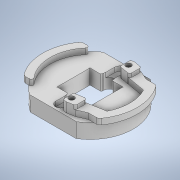
# Autodesk Inventor part: sketch01
Saved by Autodesk Inventor 2020 (Build 240168000, 168)
## iProperties
Created: 2024-03-18
Part Number: sketch01
Material: Типовые
Document SubType Name: Modeling
Designer: 4s
Density: 1 g/cm^3
Appearance: По умолчанию
Author: 4s
Autodesk Inventor part; units mm, degrees
ref_plane "YZ Plane" through (0, 0, 0) normal (1, 0, 0) x (0, 1, 0)
ref_plane "XZ Plane" through (0, 0, 0) normal (0, 1, 0) x (-1, 0, 0)
ref_plane "XY Plane" through (0, 0, 0) normal (0, 0, 1) x (1, 0, 0)
sketch "Эскиз1" plane through (0, 0, 0) normal (0, 1, 0) x (-1, 0, 0)
  line L0 (8.55, 8.55) -> (2.65, 8.55)
  line L1 (-8.55, 8.55) -> (-8.55, -8.55)
  line L2 (-8.55, -8.55) -> (-2.65, -8.55)
  line L3 (8.55, -8.55) -> (8.55, 8.55)
  line L4 (0, 0) -> (14.8515, 0) construction
  line L5 (0, 0) -> (0, -24.3542) construction
  line L6 (12.9542, 12.5) -> (-4.4938, 12.5) construction
  line L7 (12.9542, -12.5) -> (-4.4938, -12.5) construction
  arc A0 (2.65, 9.85) -> (-2.65, 9.85) centre (0, 9.85) ccw
  line L8 (2.65, 9.85) -> (2.65, 8.55)
  line L9 (-2.65, 9.85) -> (-2.65, 8.55)
  arc A1 (2.3092, 8.55) -> (2.65, 9.85) centre (0, 9.85) ccw construction
  arc A2 (-2.3092, 8.55) -> (2.3092, 8.55) centre (0, 9.85) ccw construction
  arc A3 (-2.65, 9.85) -> (-2.3092, 8.55) centre (0, 9.85) ccw construction
  line L10 (2.65, 8.55) -> (-2.65, 8.55) construction
  line L11 (-2.65, 8.55) -> (-8.55, 8.55)
  arc A4 (-2.65, -9.85) -> (2.65, -9.85) centre (0, -9.85) ccw
  line L12 (2.65, -9.85) -> (2.65, -8.55)
  line L13 (-2.65, -9.85) -> (-2.65, -8.55)
  arc A5 (2.65, -9.85) -> (2.3092, -8.55) centre (0, -9.85) ccw construction
  arc A6 (-2.3092, -8.55) -> (-2.65, -9.85) centre (0, -9.85) ccw construction
  line L14 (2.65, -8.55) -> (8.55, -8.55)
  line L15 (-2.65, -8.55) -> (2.65, -8.55) construction
  circle A7 centre (0, 0) radius 22.35
  dimension "d0" = 17.1
  dimension "d1" = 17.1
  dimension "d2" = 25
  dimension "d3" = 5.3
  dimension "d4" = 44.7
  constraints: 32 end point, 14 point on circle, 11 symmetric about line, 10 parallel, 8 centre point, 6 tangent, 5 horizontal, 5 point on line, 3 perpendicular, 2 vertical, 1 coincident, 5 other
  measures "d0" distance of L3.start L0.start
  measures "d1" distance of L1.end L3.start
  measures "d2" distance between parallel lines of L6 L7
  measures "d3" diameter of A0
  measures "d4" diameter of A7
extrude "Выдавливание1" add sketch "Эскиз1" along normal blind 7.7
sketch "Эскиз2" plane through (0, 7.7, 0) normal (0, 1, 0) x (1, 0, 0)
  line L0 (0, 0) -> (0, 23.6415) construction
  arc A0 (0, 12.825) -> (2.5, 15.325) centre (0, 15.325) ccw construction
  line L1 (0, 0) -> (14.5442, 0) construction
  arc A1 (-2.5, -15.325) -> (2.5, -15.325) centre (0, -15.325) ccw
  line L2 (2.5, -15.325) -> (2.5, -10.7289)
  circle A2 centre (0, 0) radius 22.35 construction
  line L3 (-8.55, 8.55) -> (-2.65, 8.55) construction
  line L4 (-2.65, 8.55) -> (-2.65, 9.85) construction
  arc A3 (2.65, 9.85) -> (-2.65, 9.85) centre (0, 9.85) ccw construction
  line L5 (2.65, 9.85) -> (2.65, 8.55) construction
  line L6 (2.65, 8.55) -> (8.55, 8.55) construction
  line L7 (8.55, 8.55) -> (8.55, -8.55) construction
  line L8 (8.55, -8.55) -> (2.65, -8.55) construction
  line L9 (2.65, -8.55) -> (2.65, -9.85) construction
  arc A4 (-2.65, -9.85) -> (2.65, -9.85) centre (0, -9.85) ccw construction
  line L10 (-2.65, -9.85) -> (-2.65, -8.55) construction
  line L11 (-2.65, -8.55) -> (-8.55, -8.55) construction
  line L12 (-8.55, -8.55) -> (-8.55, 8.55) construction
  line L13 (0, 0) -> (0, -9.85) construction
  line L14 (0, 0) -> (-8.55, 0) construction
  line L15 (-2.5, -15.325) -> (-2.5, -10.7289)
  line L16 (2.5, 15.325) -> (2.5, 10.7289)
  line L17 (-2.5, 15.325) -> (-2.5, 10.7289)
  arc A5 (2.5, -15.325) -> (-2.5, -15.325) centre (0, -15.325) ccw construction
  arc A6 (-2.5, 15.325) -> (0, 12.825) centre (0, 15.325) ccw construction
  arc A7 (2.5, 15.325) -> (-2.5, 15.325) centre (0, 15.325) ccw
  line L18 (2.5, -10.7289) -> (-2.5, -10.7289)
  line L19 (2.5, 10.7289) -> (-2.5, 10.7289)
  dimension "d7" = 5
  dimension "d8" = 30.65
  constraints: 20 end point, 11 point on circle, 7 symmetric about line, 5 centre point, 3 horizontal, 3 vertical, 2 point on line, 1 midpoint, 1 tangent, 1 other
  measures "d7" diameter of A0
  measures "d8" distance of A1.centre A0.centre
extrude "Выдавливание2" cut sketch "Эскиз2" against normal blind 2.5
ref_plane "РабПлоскость1" through (0, 0, -8.55) normal (-1, 0, 0) x (0, 0, 1)
sketch "Эскиз3" plane through (0, 0, -8.55) normal (-1, 0, 0) x (0, 0, 1)
  line L0 (30.9, 7.7) -> (-13.8, 7.7) construction
  line L1 (30.9, 0) -> (-13.8, 0) construction
  line L2 (30.9, 0) -> (-13.8, 0) construction
  line L3 (30.9, 0) -> (31.1, 7.7)
  line L4 (30.9, 7.7) -> (-13.8, 7.7) construction
  line L5 (31.1, 7.7) -> (30.9, 7.7)
  line L6 (30.9, 7.7) -> (30.9, 0)
  line L7 (30.9, 0) -> (30.9, 7.7) construction
  line L8 (8.55, -1.54) -> (8.55, 9.24) projected
  point P0 (8.55, 0)
  dimension "d11" = 0.2
  constraints: 6 end point, 1 collinear, 1 horizontal, 1 point on line
  measures "d11" distance of L3.end L0.start
revolve "Вращение1" add sketch "Эскиз3" angle 360 about axis through (0, 0, 0) along (0, 1, 0)
sketch "Эскиз4" plane through (0, 7.7, 0) normal (0, 1, 0) x (1, 0, 0)
  circle A0 centre (0, 0) radius 22.55 construction
  line L0 (2.5, 15.325) -> (2.5, 10.7289) construction
  arc A1 (2.65, 9.85) -> (2.5, 10.7289) centre (0, 9.85) ccw construction
  line L1 (2.65, 9.85) -> (2.65, 8.55) construction
  line L2 (2.65, 8.55) -> (8.55, 8.55) construction
  line L3 (8.55, 8.55) -> (8.55, -8.55) construction
  line L4 (8.55, -8.55) -> (2.65, -8.55) construction
  line L5 (2.65, -8.55) -> (2.65, -9.85) construction
  arc A2 (2.5, -10.7289) -> (2.65, -9.85) centre (0, -9.85) ccw construction
  line L6 (2.5, -10.7289) -> (2.5, -15.325) construction
  arc A3 (-2.5, -15.325) -> (2.5, -15.325) centre (0, -15.325) ccw construction
  line L7 (-2.5, -15.325) -> (-2.5, -10.7289) construction
  arc A4 (-2.65, -9.85) -> (-2.5, -10.7289) centre (0, -9.85) ccw construction
  line L8 (-2.65, -9.85) -> (-2.65, -8.55) construction
  line L9 (-2.65, -8.55) -> (-8.55, -8.55) construction
  line L10 (-8.55, -8.55) -> (-8.55, 8.55) construction
  line L11 (-8.55, 8.55) -> (-2.65, 8.55) construction
  line L12 (-2.65, 8.55) -> (-2.65, 9.85) construction
  arc A5 (-2.5, 10.7289) -> (-2.65, 9.85) centre (0, 9.85) ccw construction
  line L13 (-2.5, 10.7289) -> (-2.5, 15.325) construction
  arc A6 (2.5, 15.325) -> (-2.5, 15.325) centre (0, 15.325) ccw construction
  circle A7 centre (0, 0) radius 24.4 construction
  line L14 (-25.2679, -15) -> (28.9131, -15) construction
  line L15 (0, 0) -> (22.55, 0) construction
  line L16 (-25.2679, 15) -> (28.9131, 15) construction
  arc A8 (-19.2447, 15) -> (-19.2447, -15) centre (0, 0) ccw
  circle A9 centre (0, 0) radius 22.55 construction
  arc A10 (-16.8375, 15) -> (-16.8375, -15) centre (0, 0) ccw
  line L17 (-16.8375, 15) -> (-19.2447, 15)
  line L18 (-16.8375, -15) -> (-19.2447, -15)
  line L19 (0, 0) -> (0, 9.85) construction
  arc A11 (19.2447, -15) -> (19.2447, 15) centre (0, 0) ccw
  arc A12 (16.8375, -15) -> (16.8375, 15) centre (0, 0) ccw
  line L20 (16.8375, 15) -> (19.2447, 15)
  line L21 (16.8375, -15) -> (19.2447, -15)
  circle A13 centre (0, 0) radius 20.55 construction
  arc A14 (-14.0464, 15) -> (-14.0464, -15) centre (0, 0) ccw
  line L22 (-16.8375, -15) -> (-14.0464, -15)
  line L23 (-16.8375, 15) -> (-14.0464, 15)
  arc A15 (16.8375, -15) -> (16.8375, 15) centre (0, 0) ccw
  arc A16 (14.0464, -15) -> (14.0464, 15) centre (0, 0) ccw
  line L24 (16.8375, -15) -> (14.0464, -15)
  line L25 (16.8375, 15) -> (14.0464, 15)
  dimension "d13" = 1.85
  dimension "d14" = 30
  dimension "d15" = 2
  constraints: 24 end point, 20 point on circle, 9 centre point, 8 symmetric about line, 6 point on line, 4 collinear, 3 coincident, 2 concentric, 2 horizontal, 1 horizontal alignment, 1 vertical, 5 other
  measures "d14" distance between parallel lines of L14 L16
  measures "d15" radial gap between concentric circles of A9 A13
extrude "Выдавливание3" add sketch "Эскиз4" along normal blind 3
sketch "Эскиз5" plane through (0, 7.7, 0) normal (0, 1, 0) x (1, 0, 0)
  line L0 (-19.0815, -19) -> (24.7344, -19)
  line L1 (0, 0) -> (-21.0145, 0) construction
  line L2 (-19.0815, 19) -> (24.7344, 19)
  line L3 (-19.0815, -19) -> (0, -30.6052)
  line L4 (0, -30.6052) -> (24.7344, -19)
  line L5 (-19.0815, 19) -> (0, 30.6052)
  line L6 (0, 30.6052) -> (24.7344, 19)
  dimension "d18" = 38
  constraints: 14 end point, 3 symmetric about line, 2 horizontal
  measures "d18" distance between parallel lines of L0 L2
extrude "Выдавливание4" cut sketch "Эскиз5" against normal blind 10
sketch "Эскиз6" plane through (0, 0, 0) normal (0, -1, 0) x (1, 0, 0)
  line L0 (-8.55, -8.55) -> (-2.65, -8.55) construction
  line L1 (-8.55, 8.55) -> (-8.55, -8.55) construction
  line L2 (-2.65, 8.55) -> (-8.55, 8.55) construction
  line L3 (-2.65, 9.85) -> (-2.65, 8.55) construction
  arc A0 (2.65, 9.85) -> (-2.65, 9.85) centre (0, 9.85) ccw construction
  line L4 (2.65, 8.55) -> (2.65, 9.85) construction
  line L5 (8.55, 8.55) -> (2.65, 8.55) construction
  line L6 (8.55, -8.55) -> (8.55, 8.55) construction
  line L7 (2.65, -8.55) -> (8.55, -8.55) construction
  line L8 (2.65, -9.85) -> (2.65, -8.55) construction
  arc A1 (-2.65, -9.85) -> (2.65, -9.85) centre (0, -9.85) ccw construction
  line L9 (-2.65, -8.55) -> (-2.65, -9.85) construction
  line L10 (11.7696, 19) -> (-11.7696, 19) construction
  arc A2 (-11.7696, 19) -> (-11.7696, -19) centre (0, 0) ccw construction
  line L11 (-11.7696, -19) -> (11.7696, -19) construction
  arc A3 (11.7696, -19) -> (11.7696, 19) centre (0, 0) ccw construction
  line L12 (0, 9.85) -> (0, -9.85) construction
  line L13 (5.2, 15.6144) -> (5.2, -19.2684) construction
  circle A4 centre (5.2, 14.73) radius 3
  line L14 (0, 0) -> (12.7477, 0) construction
  circle A5 centre (5.2, -14.73) radius 3
  dimension "d21" = 5.2
  dimension "d22" = 6
  dimension "d23" = 29.46
  constraints: 6 end point, 2 centre point, 1 horizontal, 1 parallel, 1 point on line, 1 symmetric about line, 1 vertical, 1 other
  measures "d21" distance between parallel lines of L12 L13
  measures "d22" diameter of A4
  measures "d23" distance of A5.centre A4.centre
extrude "Выдавливание5" cut sketch "Эскиз6" against normal blind 10
sketch "Эскиз7" plane through (0, 0, 0) normal (0, -1, 0) x (1, 0, 0)
  line L0 (0, 0) -> (0, -17.2955) construction
  line L1 (9.5, 17) -> (9.5, -18.6283) construction
  line L2 (9.5, 17) -> (15.5, 13.5359)
  circle A0 centre (5.2, -14.73) radius 3 construction
  circle A1 centre (5.2, 14.73) radius 3 construction
  line L3 (-8.55, -8.55) -> (-2.65, -8.55) construction
  line L4 (-8.55, 8.55) -> (-8.55, -8.55) construction
  line L5 (-2.65, 8.55) -> (-8.55, 8.55) construction
  line L6 (-2.65, 9.85) -> (-2.65, 8.55) construction
  arc A2 (2.65, 9.85) -> (-2.65, 9.85) centre (0, 9.85) ccw construction
  line L7 (2.65, 8.55) -> (2.65, 9.85) construction
  line L8 (8.55, 8.55) -> (2.65, 8.55) construction
  line L9 (8.55, -8.55) -> (8.55, 8.55) construction
  line L10 (2.65, -8.55) -> (8.55, -8.55) construction
  line L11 (2.65, -9.85) -> (2.65, -8.55) construction
  arc A3 (-2.65, -9.85) -> (2.65, -9.85) centre (0, -9.85) ccw construction
  line L12 (-2.65, -8.55) -> (-2.65, -9.85) construction
  line L13 (11.7696, 19) -> (-11.7696, 19) construction
  arc A4 (-11.7696, 19) -> (-11.7696, -19) centre (0, 0) ccw construction
  line L14 (-11.7696, -19) -> (11.7696, -19) construction
  arc A5 (11.7696, -19) -> (11.7696, 19) centre (0, 0) ccw construction
  line L15 (15.5, 13.5359) -> (15.5, 7.5359)
  line L16 (15.5, 7.5359) -> (9.5, 11)
  line L17 (9.5, 17) -> (9.5, 11)
  line L18 (0, 0) -> (9.5, 0) construction
  line L19 (9.5, -17) -> (15.5, -13.5359)
  line L20 (15.5, -13.5359) -> (15.5, -7.5359)
  line L21 (15.5, -7.5359) -> (9.5, -11)
  line L22 (9.5, -17) -> (9.5, -11)
  dimension "d26" = 9.5
  dimension "d27" = 2
  dimension "d28" = 60
  dimension "d29" = 6
  dimension "d30" = 6
  constraints: 22 end point, 4 symmetric about line, 3 parallel, 2 point on line, 2 vertical, 1 perpendicular
  measures "d26" distance between parallel lines of L0 L1
  measures "d27" distance from line of L13 L1.start
  measures "d28" angle of L1 L2
  measures "d29" distance of L2.end L15.end
  measures "d30" distance between parallel lines of L1 L15
extrude "Выдавливание6" [suppressed]
sketch "Эскиз8" plane through (0, 7.7, 0) normal (0, 1, 0) x (1, 0, 0)
  line L0 (9.5, 24.9733) -> (9.5, -26.545) construction
  line L1 (0, -36.8486) -> (0, 35.2769) projected
  line L2 (14.0464, 15) -> (16.8375, 15) projected
  line L3 (14.0464, 15) -> (9.5, 17)
  line L4 (12.1451, 19) -> (-12.1451, 19) projected
  arc A0 (14.0464, -15) -> (14.0464, 15) centre (0, 0) ccw projected
  line L5 (14.0464, -15) -> (19.2447, -15) construction
  arc A1 (19.2447, -15) -> (19.2447, 15) centre (0, 0) ccw construction
  line L6 (19.2447, 15) -> (14.0464, 15) construction
  arc A2 (2.5, 13.4223) -> (2.4346, 15.893) centre (5.2, 14.73) ccw construction
  line L7 (2.5, 13.4223) -> (2.5, 10.7289) construction
  arc A3 (2.65, 9.85) -> (2.5, 10.7289) centre (0, 9.85) ccw construction
  line L8 (2.65, 9.85) -> (2.65, 8.55) construction
  line L9 (2.65, 8.55) -> (8.55, 8.55) construction
  line L10 (8.55, 8.55) -> (8.55, -8.55) construction
  line L11 (8.55, -8.55) -> (2.65, -8.55) construction
  line L12 (2.65, -8.55) -> (2.65, -9.85) construction
  arc A4 (2.5, -10.7289) -> (2.65, -9.85) centre (0, -9.85) ccw construction
  line L13 (2.5, -10.7289) -> (2.5, -13.4223) construction
  arc A5 (2.4346, -15.893) -> (2.5, -13.4223) centre (5.2, -14.73) ccw construction
  arc A6 (-2.5, -15.325) -> (2.4346, -15.893) centre (0, -15.325) ccw construction
  line L14 (-2.5, -15.325) -> (-2.5, -10.7289) construction
  arc A7 (-2.65, -9.85) -> (-2.5, -10.7289) centre (0, -9.85) ccw construction
  line L15 (-2.65, -9.85) -> (-2.65, -8.55) construction
  line L16 (-2.65, -8.55) -> (-8.55, -8.55) construction
  line L17 (-8.55, -8.55) -> (-8.55, 8.55) construction
  line L18 (-8.55, 8.55) -> (-2.65, 8.55) construction
  line L19 (-2.65, 8.55) -> (-2.65, 9.85) construction
  arc A8 (-2.5, 10.7289) -> (-2.65, 9.85) centre (0, 9.85) ccw construction
  line L20 (-2.5, 10.7289) -> (-2.5, 15.325) construction
  arc A9 (2.4346, 15.893) -> (-2.5, 15.325) centre (0, 15.325) ccw construction
  line L21 (-12.1451, -19) -> (12.1451, -19) construction
  arc A10 (12.1451, -19) -> (16.8375, -15) centre (0, 0) ccw construction
  line L22 (16.8375, -15) -> (14.0464, -15) construction
  arc A11 (14.0464, -15) -> (14.0464, 15) centre (0, 0) ccw construction
  line L23 (14.0464, 15) -> (16.8375, 15) construction
  arc A12 (16.8375, 15) -> (12.1451, 19) centre (0, 0) ccw construction
  line L24 (12.1451, 19) -> (-12.1451, 19) construction
  arc A13 (-12.1451, 19) -> (-16.8375, 15) centre (0, 0) ccw construction
  line L25 (-16.8375, 15) -> (-14.0464, 15) construction
  arc A14 (-14.0464, 15) -> (-14.0464, -15) centre (0, 0) ccw construction
  line L26 (-14.0464, -15) -> (-16.8375, -15) construction
  arc A15 (-16.8375, -15) -> (-12.1451, -19) centre (0, 0) ccw construction
  arc A16 (-14.0464, 15) -> (-14.0464, -15) centre (0, 0) ccw construction
  arc A17 (-16.8375, 15) -> (-16.8375, -15) centre (0, 0) ccw construction
  line L27 (-14.0464, 15) -> (-19.2447, 15) construction
  arc A18 (-19.2447, 15) -> (-19.2447, -15) centre (0, 0) ccw construction
  line L28 (-19.2447, -15) -> (-14.0464, -15) construction
  arc A19 (-14.0464, 15) -> (-14.0464, -15) centre (0, 0) ccw construction
  line L29 (9.5, 11) -> (18.244, 9.4582)
  arc A20 (14.0464, -15) -> (14.0464, 15) centre (0, 0) ccw construction
  line L30 (9.5, 17) -> (9.5, 11)
  line L31 (0, 0) -> (9.5, 0) construction
  line L32 (14.0464, -15) -> (9.5, -17)
  line L33 (9.5, -11) -> (18.244, -9.4582)
  line L34 (9.5, -17) -> (9.5, -11)
  point P0 (0, 0)
  point P1 (14.0464, 15)
  point P2 (14.0464, -15)
  dimension "d33" = 9.5
  dimension "d34" = 2
  dimension "d35" = 80
  dimension "d36" = 6
  constraints: 16 end point, 4 symmetric about line, 3 point on line, 1 collinear, 1 parallel, 1 perpendicular, 1 point on circle
  measures "d33" distance between parallel lines of L1 L0
  measures "d34" distance from line of L4 L3.end
  measures "d35" angle of L0 L29
  measures "d36" distance of L3.end L29.start
extrude "Выдавливание7" add sketch "Эскиз8" along normal blind 2
sketch "Эскиз9" plane through (0, 9.7, 0) normal (0, 1, 0) x (1, 0, 0)
  line L0 (18.244, -9.4582) -> (9.5, -11) projected
  line L1 (9.5, -11) -> (9.5, -17) projected
  line L2 (9.5, -17) -> (14.0464, -15) projected
  line L3 (9.5, 17) -> (9.5, 11) construction
  line L4 (9.5, 11) -> (18.244, 9.4582) projected
  line L5 (14.0464, 15) -> (9.5, 17) projected
  arc A0 (2.5, 13.4223) -> (2.4346, 15.893) centre (5.2, 14.73) ccw construction
  arc A1 (2.4346, -15.893) -> (2.5, -13.4223) centre (5.2, -14.73) ccw construction
  circle A2 centre (5.2, 14.73) radius 1.4
  arc A3 (5.7347, 17.682) -> (4.7237, 11.7681) centre (5.2, 14.73) ccw
  line L6 (9.5, 17) -> (5.7347, 17.682)
  line L7 (9.5, 17) -> (9.5, 11) projected
  line L8 (9.5, 11) -> (4.7237, 11.7681)
  arc A4 (4.7237, 11.7681) -> (5.7347, 17.682) centre (5.2, 14.73) ccw construction
  line L9 (0.1136, 0) -> (8.55, 0) construction
  line L10 (8.55, 8.55) -> (8.55, -8.55) construction
  circle A5 centre (5.2, -14.73) radius 1.4
  arc A6 (4.7237, -11.7681) -> (5.7347, -17.682) centre (5.2, -14.73) ccw
  line L11 (9.5, -17) -> (5.7347, -17.682)
  line L12 (9.5, -11) -> (4.7237, -11.7681)
  arc A7 (18.244, 9.4582) -> (14.0464, 15) centre (0, 0) ccw projected
  arc A8 (14.0464, -15) -> (18.244, -9.4582) centre (0, 0) ccw projected
  line L13 (0, 0) -> (0, 19.0303) construction
  line L14 (3.5, 17.2018) -> (3.5, 12.2582)
  line L15 (3.5, -17.2018) -> (3.5, -12.2582)
  point P0 (0, 0)
  dimension "d39" = 2.8
  dimension "d40" = 6
  dimension "d43" = 1.7
  constraints: 16 end point, 8 point on circle, 6 symmetric about line, 5 centre point, 3 coincident, 2 tangent, 1 horizontal, 1 midpoint, 1 parallel, 1 vertical, 2 other
  measures "d39" diameter of A2
  measures "d40" diameter of A3
  measures "d43" distance from line of A0.centre L14
extrude "Выдавливание8" add sketch "Эскиз9" along normal mid plane 6 contours A8 L2 L1 L0 | L1 L11 A6 L15 L12 | L7 L5 A7 L4 | L8 A3 L14 L6 L7
sketch "Эскиз10" plane through (0, 7.7, 0) normal (0, 1, 0) x (1, 0, 0)
  arc A0 (18.244, 9.4582) -> (14.0464, 15) centre (0, 0) ccw construction
  line L0 (14.0464, 15) -> (9.5, 17) construction
  line L1 (9.5, 17) -> (5.7347, 17.682) construction
  arc A1 (5.7347, 17.682) -> (3.5, 17.2018) centre (5.2, 14.73) ccw construction
  line L2 (4.7237, 11.7681) -> (9.5, 11) construction
  line L3 (9.5, 11) -> (18.244, 9.4582) construction
  circle A2 centre (5.2, 14.73) radius 1.4 construction
  line L4 (9.5, 17) -> (14.0464, 15) construction
  line L5 (14.0464, 15) -> (16.8375, 15) construction
  arc A3 (16.8375, 15) -> (12.1451, 19) centre (0, 0) ccw construction
  line L6 (12.1451, 19) -> (-12.1451, 19) construction
  arc A4 (-12.1451, 19) -> (-16.8375, 15) centre (0, 0) ccw construction
  line L7 (-16.8375, 15) -> (-14.0464, 15) construction
  arc A5 (-14.0464, 15) -> (-14.0464, -15) centre (0, 0) ccw construction
  line L8 (-14.0464, -15) -> (-16.8375, -15) construction
  arc A6 (-16.8375, -15) -> (-12.1451, -19) centre (0, 0) ccw construction
  line L9 (-12.1451, -19) -> (12.1451, -19) construction
  arc A7 (12.1451, -19) -> (16.8375, -15) centre (0, 0) ccw construction
  line L10 (16.8375, -15) -> (14.0464, -15) construction
  line L11 (14.0464, -15) -> (9.5, -17) construction
  line L12 (9.5, -11) -> (18.244, -9.4582) construction
  arc A8 (18.244, -9.4582) -> (18.244, 9.4582) centre (0, 0) ccw construction
  line L13 (18.244, 9.4582) -> (9.5, 11) construction
  arc A9 (3.5, 17.2018) -> (2.4346, 15.893) centre (5.2, 14.73) ccw construction
  line L14 (2.5, 13.4223) -> (2.5, 10.7289) construction
  arc A10 (2.65, 9.85) -> (2.5, 10.7289) centre (0, 9.85) ccw construction
  line L15 (2.65, 9.85) -> (2.65, 8.55) construction
  line L16 (2.65, 8.55) -> (8.55, 8.55) construction
  line L17 (8.55, 8.55) -> (8.55, -8.55) construction
  line L18 (8.55, -8.55) -> (2.65, -8.55) construction
  line L19 (2.65, -8.55) -> (2.65, -9.85) construction
  arc A11 (2.5, -10.7289) -> (2.65, -9.85) centre (0, -9.85) ccw construction
  line L20 (2.5, -10.7289) -> (2.5, -13.4223) construction
  arc A12 (3.5, -12.2582) -> (2.5, -13.4223) centre (5.2, -14.73) ccw construction
  arc A13 (-2.5, -15.325) -> (2.4346, -15.893) centre (0, -15.325) ccw construction
  line L21 (-2.5, -15.325) -> (-2.5, -10.7289) construction
  arc A14 (-2.65, -9.85) -> (-2.5, -10.7289) centre (0, -9.85) ccw construction
  line L22 (-2.65, -9.85) -> (-2.65, -8.55) construction
  line L23 (-2.65, -8.55) -> (-8.55, -8.55) construction
  line L24 (-8.55, -8.55) -> (-8.55, 8.55) construction
  line L25 (-8.55, 8.55) -> (-2.65, 8.55) construction
  line L26 (-2.65, 8.55) -> (-2.65, 9.85) construction
  arc A15 (-2.5, 10.7289) -> (-2.65, 9.85) centre (0, 9.85) ccw construction
  line L27 (-2.5, 10.7289) -> (-2.5, 15.325) construction
  arc A16 (2.4346, 15.893) -> (-2.5, 15.325) centre (0, 15.325) ccw construction
  arc A17 (3.5, 12.2582) -> (4.7237, 11.7681) centre (5.2, 14.73) ccw projected
  line L28 (3.5, 17.2018) -> (3.5, 12.2582) projected
  line L29 (5.7347, 17.682) -> (9.5, 17) projected
  line L30 (9.5, -17) -> (5.7347, -17.682) projected
  arc A18 (3.5, -17.2018) -> (5.7347, -17.682) centre (5.2, -14.73) ccw projected
  arc A19 (2.4346, -15.893) -> (3.5, -17.2018) centre (5.2, -14.73) ccw projected
  arc A20 (5.7347, 17.682) -> (3.5, 17.2018) centre (5.2, 14.73) ccw projected
  line L31 (9.5, 11) -> (4.7237, 11.7681) projected
  arc A21 (3.5, 12.2582) -> (4.7237, 11.7681) centre (5.2, 14.73) ccw projected
  arc A22 (2.5, 13.4223) -> (3.5, 12.2582) centre (5.2, 14.73) ccw projected
  arc A23 (4.7237, -11.7681) -> (3.5, -12.2582) centre (5.2, -14.73) ccw projected
  line L32 (4.7237, -11.7681) -> (9.5, -11) projected
  point P0 (0, 0)
sketch "Эскиз11" plane through (0, 7.7, 0) normal (0, 1, 0) x (1, 0, 0)
  arc A0 (3.5, 17.2018) -> (2.4346, 15.893) centre (5.2, 14.73) ccw projected
  arc A1 (2.5, 13.4223) -> (3.5, 12.2582) centre (5.2, 14.73) ccw projected
  arc A2 (3.5, 17.2018) -> (3.5, 12.2582) centre (5.2, 14.73) ccw
  circle A3 centre (5.2, 14.73) radius 1.4 construction
  line L0 (0, 0) -> (8.55, 0) construction
  line L1 (8.55, 8.55) -> (8.55, -8.55) construction
  arc A4 (3.5, -12.2582) -> (3.5, -17.2018) centre (5.2, -14.73) ccw
  line L2 (3.5, 17.2018) -> (3.5, 12.2582) projected
  line L3 (3.5, 17.2018) -> (3.5, 12.2582)
  arc A5 (3.5, -12.2582) -> (2.5, -13.4223) centre (5.2, -14.73) ccw projected
  arc A6 (2.4346, -15.893) -> (3.5, -17.2018) centre (5.2, -14.73) ccw projected
  line L4 (3.5, -12.2582) -> (3.5, -17.2018)
  point P0 (2.5, 13.4223)
  constraints: 6 end point, 4 point on circle, 3 symmetric about line, 2 centre point, 1 coincident, 1 collinear, 1 midpoint, 1 vertical, 1 other
extrude "Выдавливание9" add sketch "Эскиз11" against normal up to surface (1 mm away)
fillet "Сопряжение1" radius 0.5 4 edges at (3.5, 10.2, 12.2582) (3.5, 10.2, 17.2018) (3.5, 10.2, -12.2582) (3.5, 10.2, -17.2018)
fillet "Сопряжение2" radius 0.7 4 edges at (2.65, 3.85, -8.55) (2.65, 3.85, 8.55) (-2.65, 3.85, 8.55) (-2.65, 3.85, -8.55)
fillet "Сопряжение3" radius 1 4 edges at (-14.0464, 9.2, -15) (-14.0464, 9.2, 15) (18.244, 11.7, 9.4582) (18.244, 11.7, -9.4582)
sketch "Эскиз12" plane through (0, 12.7, 0) normal (0, 1, 0) x (1, 0, 0)
  arc A0 (19.2447, -15) -> (19.2447, 15) centre (0, 0) ccw construction
  line L0 (14.0464, -15) -> (19.2447, -15) construction
  arc A1 (19.2447, -15) -> (19.2447, 15) centre (0, 0) ccw construction
  line L1 (19.2447, 15) -> (14.0464, 15) construction
  arc A2 (17.1161, 11.3728) -> (14.0464, 15) centre (0, 0) ccw construction
  arc A3 (16.1096, 9.8346) -> (17.1161, 11.3728) centre (16.2832, 10.8194) ccw construction
  line L2 (16.1096, 9.8346) -> (18.244, 9.4582) construction
  arc A4 (18.244, -9.4582) -> (18.244, 9.4582) centre (0, 0) ccw construction
  line L3 (18.244, -9.4582) -> (16.1096, -9.8346) construction
  arc A5 (17.1161, -11.3728) -> (16.1096, -9.8346) centre (16.2832, -10.8194) ccw construction
  arc A6 (14.0464, -15) -> (17.1161, -11.3728) centre (0, 0) ccw construction
  circle A7 centre (5.2, -14.73) radius 1.4 construction
  arc A8 (17.1161, -11.3728) -> (16.1096, -9.8346) centre (16.2832, -10.8194) ccw construction
  line L4 (16.1096, -9.8346) -> (9.5, -11) construction
  line L5 (9.5, -11) -> (4.7237, -11.7681) construction
  arc A9 (4.7237, -11.7681) -> (3.76, -12.0982) centre (5.2, -14.73) ccw construction
  arc A10 (3.76, -12.0982) -> (3.5, -12.5368) centre (4, -12.5368) ccw construction
  line L6 (3.5, -12.5368) -> (3.5, -16.9232) construction
  arc A11 (3.5, -16.9232) -> (3.76, -17.3618) centre (4, -16.9232) ccw construction
  arc A12 (3.76, -17.3618) -> (5.7347, -17.682) centre (5.2, -14.73) ccw construction
  line L7 (5.7347, -17.682) -> (9.5, -17) construction
  line L8 (9.5, -17) -> (14.0464, -15) construction
  arc A13 (14.0464, -15) -> (17.1161, -11.3728) centre (0, 0) ccw construction
  circle A14 centre (5.2, 14.73) radius 1.4 construction
  arc A15 (16.1096, 9.8346) -> (17.1161, 11.3728) centre (16.2832, 10.8194) ccw construction
  arc A16 (17.1161, 11.3728) -> (14.0464, 15) centre (0, 0) ccw construction
  line L9 (14.0464, 15) -> (9.5, 17) construction
  line L10 (9.5, 17) -> (5.7347, 17.682) construction
  arc A17 (5.7347, 17.682) -> (3.76, 17.3618) centre (5.2, 14.73) ccw construction
  arc A18 (3.76, 17.3618) -> (3.5, 16.9232) centre (4, 16.9232) ccw construction
  line L11 (3.5, 16.9232) -> (3.5, 12.5368) construction
  arc A19 (3.5, 12.5368) -> (3.76, 12.0982) centre (4, 12.5368) ccw construction
  arc A20 (3.76, 12.0982) -> (4.7237, 11.7681) centre (5.2, 14.73) ccw construction
  line L12 (4.7237, 11.7681) -> (9.5, 11) construction
  line L13 (9.5, 11) -> (16.1096, 9.8346) construction
  line L14 (9.5, 17) -> (9.5, 11)
  line L15 (9.5, 17) -> (14.0464, 15) projected
  line L16 (9.5, 17) -> (13.9034, 16.6477)
  line L17 (13.9034, 16.6477) -> (18.109, 11.384)
  line L18 (18.109, 11.384) -> (17.6433, 7.6267)
  line L19 (17.6433, 7.6267) -> (9.5, 11)
  line L20 (0, 0) -> (20.55, 0) construction
  arc A21 (18.244, -9.4582) -> (18.244, 9.4582) centre (0, 0) ccw construction
  arc A22 (14.0464, -15) -> (17.1161, -11.3728) centre (0, 0) ccw construction
  arc A23 (17.1161, -11.3728) -> (16.1096, -9.8346) centre (16.2832, -10.8194) ccw construction
  line L21 (16.1096, -9.8346) -> (18.244, -9.4582) construction
  arc A24 (17.1161, -11.3728) -> (16.1096, -9.8346) centre (16.2832, -10.8194) ccw construction
  arc A25 (14.0464, -15) -> (17.1161, -11.3728) centre (0, 0) ccw construction
  line L22 (14.0464, -15) -> (9.5, -17) construction
  line L23 (9.5, -11) -> (16.1096, -9.8346) construction
  line L24 (9.5, -17) -> (9.5, -11)
  line L25 (9.5, -17) -> (14.0464, -15)
  line L26 (9.5, -17) -> (13.9034, -16.6477)
  line L27 (13.9034, -16.6477) -> (18.109, -11.384)
  line L28 (18.109, -11.384) -> (17.6433, -7.6267)
  line L29 (17.6433, -7.6267) -> (9.5, -11)
  point P0 (0, 0)
  constraints: 30 end point, 14 symmetric about line, 10 point on circle, 4 centre point, 1 vertical, 4 other
extrude "Выдавливание10" cut sketch "Эскиз12" against normal up to surface (2 mm away)
fillet "Сопряжение4" radius 1 4 edges at (9.5, 11.7, 11) (9.5, 11.7, 17) (9.5, 11.7, -11) (9.5, 11.7, -17)
fillet "Сопряжение5" radius 2 4 edges at (-19.2447, 9.2, -15) (-19.2447, 9.2, 15) (19.2447, 9.2, 15) (19.2447, 9.2, -15)
